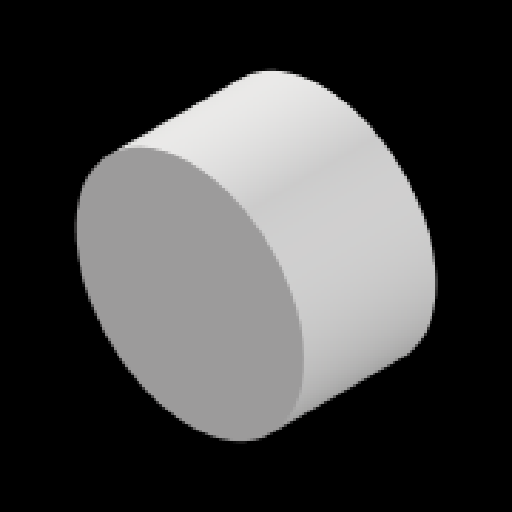
# Autodesk Inventor part: BackCapV1
Saved by Autodesk Inventor 2024 (Build 280153000, 153)
## iProperties
Created: 2026-04-10
Part Number: BackCapV1
Material: Generic
Document SubType Name: Modeling
Designer: Tanner
Density: 1 g/cm^3
Appearance: Default
Author: Tanner
Autodesk Inventor part; units mm, degrees
ref_plane "YZ Plane" through (0, 0, 0) normal (1, 0, 0) x (0, 1, 0)
ref_plane "XZ Plane" through (0, 0, 0) normal (0, 1, 0) x (-1, 0, 0)
ref_plane "XY Plane" through (0, 0, 0) normal (0, 0, 1) x (1, 0, 0)
sketch "Sketch1" plane through (0, 0, 0) normal (1, 0, 0) x (0, 1, 0)
  line L0 (106.6, 0) -> (106.6, -254) construction
  line L1 (101.6, -254) -> (101.6, 0) construction
  line L2 (-106.6, 0) -> (106.6, 0) construction
  line L3 (107.1, 0) -> (107.1, -30)
  line L4 (107.1, -30) -> (112.1, -30)
  line L5 (112.1, -30) -> (112.1, 100)
  line L6 (112.1, 100) -> (0, 100)
  line L7 (107.1, 0) -> (97.1, 0)
  line L8 (97.1, 0) -> (97.1, 90)
  line L9 (97.1, 90) -> (0, 90)
  line L10 (0, 90) -> (0, 100)
  point P0 (0, 0)
  point P1 (0, 0)
  dimension "d2" = 5
  dimension "d4" = 0.5
  dimension "d5" = 30
  dimension "d6" = 100
  dimension "d8" = 10
  dimension "d9" = 10
  constraints: 20 end point, 4 perpendicular, 4 vertical, 1 horizontal, 1 horizontal alignment, 1 midpoint, 1 point on line, 1 vertical alignment, 4 other
  measures "d2" distance between parallel lines of L3 L5
  measures "d4" distance between parallel lines of L3 L0
  measures "d5" distance between parallel lines of L2 L4
  measures "d6" distance between parallel lines of L6 L2
  measures "d8" distance of L3.start L7.end
  measures "d9" distance between parallel lines of L6 L9
revolve "Revolution1" add sketch "Sketch1" angle 360 about axis through (0, 0, 90) along (0, 0, 1)
body "Solid1"
